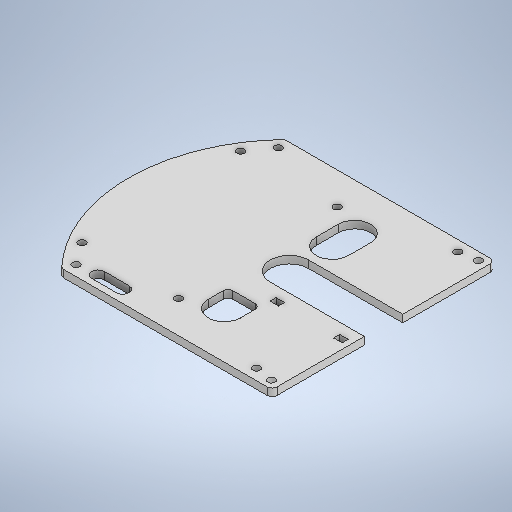
# Autodesk Inventor part: base_nivel2
Saved by Autodesk Inventor 2025.2 (Build 292293000, 293)
## iProperties
Created: 2025-04-02
Part Number: base_nivel2
Material: Generic
Document SubType Name: Modeling
Designer: cdavi
Density: 1 g/cm^3
Appearance: Default
Author: cdavi
Autodesk Inventor part; units mm, degrees
ref_plane "YZ Plane" through (0, 0, 0) normal (1, 0, 0) x (0, 1, 0)
ref_plane "XZ Plane" through (0, 0, 0) normal (0, 1, 0) x (-1, 0, 0)
ref_plane "XY Plane" through (0, 0, 0) normal (0, 0, 1) x (1, 0, 0)
sketch "Sketch1" plane through (0, 0, 0) normal (0, 1, 0) x (-1, 0, 0)
  circle A0 centre (0, 0) radius 54.1913 construction
  line L0 (0, 54.1913) -> (0, -54.1913) construction
  circle A1 centre (-34.5, 41.7906) radius 1.5
  line L1 (0, 0) -> (-54.1913, 0)
  circle A2 centre (-34.5, -41.7906) radius 1.5
  line L2 (-38, 52.7352) -> (-38, -52.7352)
  circle A3 centre (0, 0) radius 7.75
  line L3 (0, 7.75) -> (-38, 7.75)
  line L4 (0, -7.75) -> (-38, -7.75)
  circle A4 centre (0, 0) radius 65
  circle A5 centre (-34.5, -41.7906) radius 1.5
  line L5 (12.75, 32) -> (51.75, 32) construction
  line L6 (51.75, 32) -> (51.75, -32) construction
  line L7 (51.75, -32) -> (12.75, -32) construction
  line L8 (12.75, -32) -> (12.75, 32) construction
  circle A6 centre (0, 0) radius 70 construction
  line L9 (-45, 53.619) -> (-45, -53.619) construction
  line L10 (0, 0) -> (-34.5, 41.7906) construction
  circle A7 centre (-27.3, 40.619) radius 1.5
  circle A8 centre (-27.3, -40.619) radius 1.5
  circle A9 centre (51.75, -32) radius 1.5
  line L11 (51.75, -32) -> (55.2843, -34.1855)
  circle A10 centre (51.75, 32) radius 1.5
  circle A11 centre (12.75, 32) radius 1.5
  circle A12 centre (12.75, -32) radius 1.5
  circle A13 centre (45.3318, 40.817) radius 1.5
  circle A14 centre (45.3318, -40.817) radius 1.5
  line L12 (-6.6, 12.025) -> (-10, 12.025)
  line L13 (-10, 12.025) -> (-10, 14.425)
  line L14 (-10, 14.425) -> (-6.6, 14.425)
  line L15 (-6.6, 14.425) -> (-6.6, 12.025)
  line L16 (0, 26.3) -> (0, 17.3) construction
  line L17 (-6.5, 26.3) -> (-6.5, 17.3)
  line L18 (6.5, 17.3) -> (6.5, 26.3)
  arc A15 (6.5, 26.3) -> (-6.5, 26.3) centre (0, 26.3) ccw
  arc A16 (-6.5, 17.3) -> (6.5, 17.3) centre (0, 17.3) ccw
  line L19 (-6.5, -26.3) -> (-6.5, -17.3)
  line L20 (6.5, -17.3) -> (6.5, -26.3)
  arc A17 (-6.5, -26.3) -> (6.5, -26.3) centre (0, -26.3) ccw
  arc A18 (6.5, -17.3) -> (-6.5, -17.3) centre (0, -17.3) ccw
  line L21 (0, 0) -> (-12.842, 0) construction
  line L22 (-10, 12.025) -> (-26.65, 12.025) construction
  line L23 (-26.65, 12.025) -> (-26.65, 0) construction
  line L24 (-26.65, 0) -> (-17.65, 0)
  line L25 (0, 0) -> (45.3318, 40.817) construction
  line L26 (-8.3, 12.025) -> (-27.425, 12.025) construction
  line L27 (-27.425, 12.025) -> (-27.425, 0) construction
  line L28 (-7.75, 0) -> (-11.25, 0)
  line L29 (-11.25, 0) -> (-15.25, 0)
  line L30 (6.5, 18.3) -> (-6.5, 18.3)
  line L31 (-32.35, 12.025) -> (-35.75, 12.025)
  line L32 (-35.75, 12.025) -> (-35.75, 14.425)
  line L33 (-35.75, 14.425) -> (-32.35, 14.425)
  line L34 (-32.35, 14.425) -> (-32.35, 12.025)
  line L35 (37.25, 40) -> (27.25, 40) construction
  line L36 (37.25, 42.5) -> (27.25, 42.5)
  line L37 (27.25, 37.5) -> (37.25, 37.5)
  arc A19 (37.25, 37.5) -> (37.25, 42.5) centre (37.25, 40) ccw
  arc A20 (27.25, 42.5) -> (27.25, 37.5) centre (27.25, 40) ccw
  line L38 (46.9042, -45) -> (-38, -45)
  line L39 (46.9042, 45) -> (-38, 45)
  line L40 (-6.5, 18.3) -> (-6.6, 14.425) construction
  point P0 (12.75, 0)
  point P1 (7.75, 0)
  point P2 (0, -7.75)
  point P3 (-38, -7.75)
  point P4 (51.75, -16.0823)
  point P5 (51.75, -30.5)
  point P6 (50.25, -32)
  point P7 (43.7344, -32)
  point P8 (51.75, 16.0823)
  point P9 (43.7344, 32)
  point P10 (50.25, 32)
  point P11 (51.75, 30.5)
  point P12 (0, 21.8)
  point P13 (0, 10.8)
  point P14 (0, 32.8)
  point P15 (-45, -46.9042)
  point P16 (-45, 46.9042)
  point P17 (52.6522, 30.8017)
  point P18 (51.081, 33.3426)
  point P19 (51.081, -33.3426)
  point P20 (52.6522, -30.8017)
  point P21 (32.25, 40)
  point P22 (32.25, 32)
  point P23 (46.9042, 45)
  point P24 (-38, 45)
  dimension "d2" = 3
  dimension "d3" = 38
  dimension "d4" = 15.5
  dimension "d5" = 130
  dimension "d6" = 39
  dimension "d7" = 64
  dimension "d8" = 5
  dimension "d9" = 140
  dimension "d11" = 45
  dimension "d15" = 108.3827
  dimension "d16" = 39.541
  dimension "d17" = 3
  dimension "d18" = 17.7
  dimension "d19" = 13
  dimension "d20" = 3
  dimension "d21" = 4.1554
  dimension "d40" = 2.4
  dimension "d41" = 3.4
  dimension "d42" = 4.275
  dimension "d43" = 28
  dimension "d45" = 13
  dimension "d46" = 22
  dimension "d49" = 21.8
  dimension "d51" = 12.842
  dimension "d52" = 16.65
  dimension "d53" = 9
  dimension "d54" = 4.808
  dimension "d56" = 4.2947
  dimension "d58" = 48
  dimension "d59" = 61
  dimension "d60" = 3
  dimension "d63" = 19.125
  dimension "d64" = 3.5
  dimension "d66" = 4
  dimension "d67" = 12.175
  dimension "d68" = 1
  dimension "d69" = 22.35
  dimension "d70" = 5
  dimension "d71" = 5.5
  dimension "d72" = 10
  dimension "d75" = 45
  dimension "d76" = 3.8763
  constraints: 86 end point, 27 point on circle, 21 centre point, 16 point on line, 13 symmetric about line, 9 coincident, 9 parallel, 9 tangent, 8 perpendicular, 7 midpoint, 5 horizontal, 3 equal radius, 3 vertical, 2 equal length, 2 horizontal alignment, 1 line through centre, 1 vertical alignment, 6 other
  measures "d2" diameter of A1
  measures "d3" distance between parallel lines of L0 L2
  measures "d4" diameter of A3
  measures "d5" diameter of A4
  measures "d6" distance between parallel lines of L8 L6
  measures "d7" distance of L5.end L6.end
  measures "d8" distance from line of A3.end L8
  measures "d9" diameter of A6
  measures "d11" distance from line of L9 A3.centre
  measures "d15" diameter of A0
  measures "d16" angle of L0 L10
  measures "d17" diameter of A7
  measures "d18" horizontal distance of L9.start A7.centre
  measures "d19" vertical distance of L9.start A7.centre
  measures "d20" diameter of A9
  measures "d21" distance of L11.start L11.end
  measures "d40" distance of L14.end L12.start
  measures "d41" distance of L13.end L14.end
  measures "d42" distance between parallel lines of L3 L12
  measures "d43" distance between parallel lines of L2 L13
  measures "d45" distance between parallel lines of L17 L18
  measures "d46" distance of point (0, 10.8) point (0, 32.8)
  measures "d49" distance of point (0, 0) point (0, 21.8)
  measures "d51" distance of point (0, 0) L21.end
  measures "d52" distance of L12.end L22.end
  measures "d53" distance of L23.end L24.end
  measures "d54" distance of L24.end L21.end
  measures "d58" angle of L0 L25
  measures "d59" distance of L21.start L25.end
  measures "d60" diameter of A13
  measures "d63" distance of L26.end L26.start
  measures "d64" distance of L28.start L28.end
  measures "d66" distance of L28.end L29.end
  measures "d67" distance of L27.end L29.end
  measures "d68" distance from line of L30 L16.end
  measures "d69" distance between parallel lines of L34 L13
  measures "d70" distance between parallel lines of L36 L37
  measures "d71" distance between parallel lines of L5 L37
  measures "d72" distance of L37.start L37.end
  measures "d75" distance from line of A4.centre L38
  measures "d76" distance of L30.end L14.end
extrude "Extrusion1" add sketch "Sketch1" along normal blind 3 contours L3 L2 L39 A4 L38 L4 A3 | L30 L18 A16 L17
fillet "Fillet1" radius 2 6 edges at (38, 1.5, 45) (38, 1.5, -45) (-46.9042, 1.5, 45) (-46.9042, 1.5, -45) (-6.5, 1.5, 18.3) (6.5, 1.5, 18.3)
fillet "Fillet2" [suppressed]
body "Solid1"
